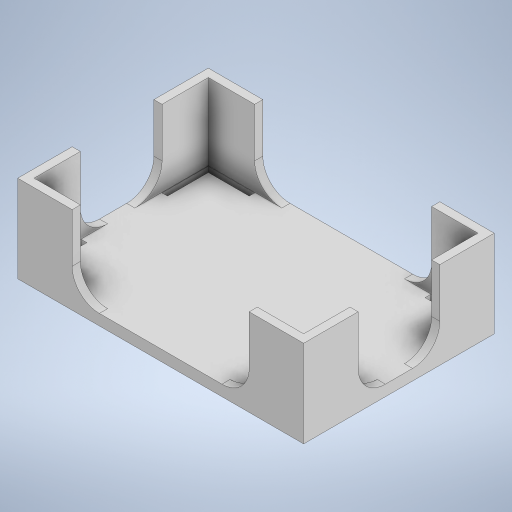
# Autodesk Inventor part: TestingPlatform_standardStack01
Saved by Autodesk Inventor 2024.2 (Build 282272000, 272)
## iProperties
Created: 2024-01-29
Part Number: TestingPlatform_standardStack01
Material: Generic
Document SubType Name: Modeling
Designer: ringl
Density: 1 g/cm^3
Appearance: Default
Author: ringl
Autodesk Inventor part; units mm, degrees
ref_plane "YZ Plane" through (0, 0, 0) normal (1, 0, 0) x (0, 1, 0)
ref_plane "XZ Plane" through (0, 0, 0) normal (0, 1, 0) x (-1, 0, 0)
ref_plane "XY Plane" through (0, 0, 0) normal (0, 0, 1) x (1, 0, 0)
sketch "Sketch1" plane through (0, 0, 0) normal (0, 1, 0) x (-1, 0, 0)
  line L0 (0, 0) -> (105, 0)
  line L1 (105, 0) -> (105, -70)
  line L2 (105, -70) -> (0, -70)
  line L3 (0, -70) -> (0, 0)
  dimension "d0" = 105
  dimension "d1" = 70
  constraints: 8 end point, 2 parallel, 1 horizontal, 1 perpendicular
  measures "d0" distance of L1.end L2.end
  measures "d1" distance of L0.end L1.end
extrude "Extrusion1" add sketch "Sketch1" along normal blind 4
sketch "Sketch2" plane through (0, 0, 0) normal (0, -1, 0) x (1, 0, 0)
  line L0 (-101.8, -3.2) -> (-84.8, -3.2)
  line L1 (-84.8, -3.2) -> (-84.8, -5.2)
  line L2 (-84.8, -5.2) -> (-99.8, -5.2)
  line L3 (-99.8, -5.2) -> (-99.8, -20.2)
  line L4 (-99.8, -20.2) -> (-101.8, -20.2)
  line L5 (-101.8, -20.2) -> (-101.8, -3.2)
  line L6 (-105, 0) -> (0, 0) projected
  line L7 (-105, -70) -> (-105, 0) projected
  line L8 (-52.5, 13.4533) -> (-52.5, -78.582) construction
  line L9 (-116.2226, -35) -> (14.8802, -35) construction
  line L10 (-3.2, -3.2) -> (-20.2, -3.2)
  line L11 (-20.2, -3.2) -> (-20.2, -5.2)
  line L12 (-20.2, -5.2) -> (-5.2, -5.2)
  line L13 (-5.2, -5.2) -> (-5.2, -20.2)
  line L14 (-5.2, -20.2) -> (-3.2, -20.2)
  line L15 (-3.2, -20.2) -> (-3.2, -3.2)
  line L16 (-101.8, -66.8) -> (-84.8, -66.8)
  line L17 (-84.8, -66.8) -> (-84.8, -64.8)
  line L18 (-84.8, -64.8) -> (-99.8, -64.8)
  line L19 (-99.8, -64.8) -> (-99.8, -49.8)
  line L20 (-99.8, -49.8) -> (-101.8, -49.8)
  line L21 (-101.8, -49.8) -> (-101.8, -66.8)
  line L22 (-3.2, -66.8) -> (-20.2, -66.8)
  line L23 (-3.2, -49.8) -> (-3.2, -66.8)
  line L24 (-5.2, -49.8) -> (-3.2, -49.8)
  line L25 (-5.2, -64.8) -> (-5.2, -49.8)
  line L26 (-20.2, -64.8) -> (-5.2, -64.8)
  line L27 (-20.2, -66.8) -> (-20.2, -64.8)
  dimension "d4" = 17
  dimension "d5" = 2
  dimension "d6" = 17
  dimension "d7" = 2
  dimension "d8" = 3.2
  dimension "d9" = 3.2
  dimension "d10" = 52.5
  dimension "d11" = 35
  constraints: 52 end point, 18 symmetric about line, 5 perpendicular, 2 horizontal, 1 vertical
  measures "d4" distance of L0.start L0.end
  measures "d5" distance of L0.end L1.end
  measures "d6" distance of L4.end L0.start
  measures "d7" distance of L3.end L4.end
  measures "d8" distance between parallel lines of L6 L0
  measures "d9" distance between parallel lines of L7 L5
  measures "d10" distance from line of L8 L6.end
  measures "d11" distance between parallel lines of L6 L9
extrude "Extrusion2" cut sketch "Sketch2" against normal through all
sketch "Sketch3" plane through (0, 4, 0) normal (0, 1, 0) x (1, 0, 0)
  line L0 (-105, 70) -> (-105, 0) projected
  line L1 (-105, 70) -> (-105, 50)
  line L2 (-105, 50) -> (-102, 50)
  line L3 (-105, 70) -> (-85, 70)
  line L4 (0, 70) -> (-105, 70) projected
  line L5 (-85, 70) -> (-85, 67)
  line L6 (-85, 67) -> (-102, 67)
  line L7 (-102, 67) -> (-102, 50)
  line L8 (-52.5, 99.9312) -> (-52.5, -17.7346) construction
  line L9 (-124.2156, 35) -> (28.5486, 35) construction
  line L10 (0, 70) -> (0, 50)
  line L11 (0, 50) -> (-3, 50)
  line L12 (0, 70) -> (-20, 70)
  line L13 (-20, 70) -> (-20, 67)
  line L14 (-20, 67) -> (-3, 67)
  line L15 (-3, 67) -> (-3, 50)
  line L16 (19.2156, 35) -> (-133.5486, 35) construction
  line L17 (-105, 0) -> (-105, 20)
  line L18 (-105, 20) -> (-102, 20)
  line L19 (-105, 0) -> (-85, 0)
  line L20 (-85, 0) -> (-85, 3)
  line L21 (-85, 3) -> (-102, 3)
  line L22 (-102, 3) -> (-102, 20)
  line L23 (-52.5, -29.9312) -> (-52.5, 87.7346) construction
  line L24 (0, 0) -> (0, 20)
  line L25 (0, 20) -> (-3, 20)
  line L26 (0, 0) -> (-20, 0)
  line L27 (-20, 0) -> (-20, 3)
  line L28 (-20, 3) -> (-3, 3)
  line L29 (-3, 3) -> (-3, 20)
  point P0 (-105, 20)
  point P1 (-20, 70)
  point P2 (0.75, 3)
  point P3 (2, 8)
  point P4 (2, 62)
  point P5 (0.75, 67)
  dimension "d15" = 20
  dimension "d16" = 3
  dimension "d17" = 20
  dimension "d18" = 3
  dimension "d19" = 52.5
  dimension "d20" = 35
  constraints: 56 end point, 20 symmetric about line, 4 perpendicular, 2 point on line, 1 horizontal, 1 vertical
  measures "d15" distance of L0.start L1.end
  measures "d16" distance of L1.end L2.end
  measures "d17" distance of L0.start L3.end
  measures "d18" distance of L3.end L5.end
  measures "d19" distance from line of point (0, 0) L8
  measures "d20" distance from line of point (0, 0) L9
extrude "Extrusion3" add sketch "Sketch3" along normal blind 28
fillet "Fillet2" radius 10 8 edges at (-85, 4, -1.5) (-20, 4, -1.5) (-1.5, 4, -20) (-103.5, 4, -20) (-1.5, 4, -50) (-103.5, 4, -50) (-85, 4, -68.5) (-20, 4, -68.5)
body "Solid1"
